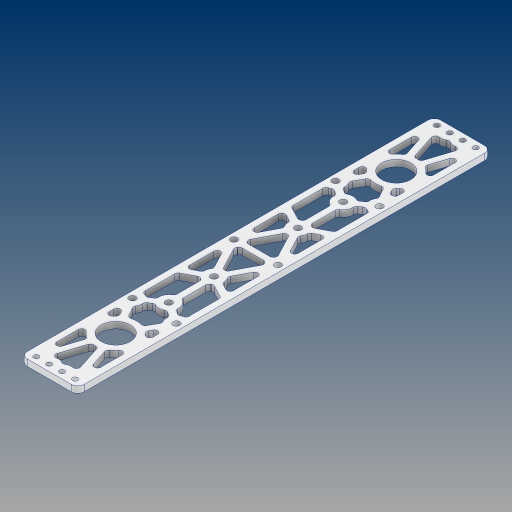
# Autodesk Inventor part: ELEV_019_SUPBAR3
Saved by Autodesk Inventor 2024.3 (Build 283343000, 343)
## iProperties
Created: 2024-11-28
Part Number: ELEV_019_SUPBAR3
Material: Aluminum 6061
Document SubType Name: Modeling
Designer: Kenji
Density: 2.7 g/cm^3
Appearance: Aluminum - Flat
Author: Kenji
Autodesk Inventor part; units mm, degrees
ref_plane "YZ Plane" through (0, 0, 0) normal (1, 0, 0) x (0, 1, 0)
ref_plane "XZ Plane" through (0, 0, 0) normal (0, 1, 0) x (-1, 0, 0)
ref_plane "XY Plane" through (0, 0, 0) normal (0, 0, 1) x (1, 0, 0)
sketch "Sketch1" plane through (0, 0, 0) normal (0, 1, 0) x (-1, 0, 0)
  line L0 (0, 0) -> (55.88, 0)
  line L1 (55.88, 0) -> (55.88, -406.4)
  line L2 (55.88, -406.4) -> (0, -406.4)
  line L3 (0, -406.4) -> (0, 0)
  circle A0 centre (27.94, -65.3034) radius 14.2875
  circle A1 centre (27.94, -341.0966) radius 14.2875
  line L4 (27.94, 0) -> (27.94, -406.4) construction
  circle A2 centre (27.94, -341.0966) radius 22.733 construction
  circle A3 centre (27.94, -65.3034) radius 22.733 construction
  circle A4 centre (27.94, -65.3034) radius 27.2288 construction
  circle A5 centre (27.94, -341.0966) radius 27.2288 construction
  circle A6 centre (27.94, -117.475) radius 3.2512
  circle A7 centre (27.94, -161.925) radius 3.2512
  circle A8 centre (27.94, -244.475) radius 3.2512
  circle A9 centre (27.94, -288.925) radius 3.2512
  line L5 (55.88, -203.2) -> (0, -203.2) construction
  line L6 (55.88, -368.3254) -> (0, -368.3254) construction
  line L7 (47.244, -254) -> (8.636, -254) construction
  line L8 (8.636, -254) -> (8.636, -279.4) construction
  line L9 (8.636, -279.4) -> (47.244, -279.4) construction
  line L10 (47.244, -279.4) -> (47.244, -254) construction
  line L11 (27.94, -254) -> (27.94, -279.4) construction
  circle A10 centre (8.89, -6.35) radius 2.54
  circle A11 centre (21.59, -6.35) radius 2.54
  circle A12 centre (34.29, -6.35) radius 2.54
  circle A13 centre (46.99, -6.35) radius 2.54
  circle A14 centre (8.89, -400.05) radius 2.54
  circle A15 centre (21.59, -400.05) radius 2.54
  circle A16 centre (34.29, -400.05) radius 2.54
  circle A17 centre (46.99, -400.05) radius 2.54
  circle A18 centre (49.53, -203.2) radius 3.2512
  circle A19 centre (49.53, -203.2) radius 6.35 construction
  circle A20 centre (6.35, -203.2) radius 3.2512
  circle A21 centre (6.35, -203.2) radius 6.35 construction
  line L12 (49.53, -203.2) -> (6.35, -203.2) construction
  circle A22 centre (49.53, -103.378) radius 3.2512
  circle A23 centre (6.35, -103.378) radius 3.2512
  circle A24 centre (49.53, -103.378) radius 6.35 construction
  circle A25 centre (6.35, -103.378) radius 6.35 construction
  line L13 (49.53, -103.378) -> (6.35, -103.378) construction
  line L14 (27.94, -103.378) -> (27.94, -92.5322) construction
  line L15 (27.94, -103.378) -> (27.94, -114.2238) construction
  circle A26 centre (49.53, -303.022) radius 3.2512
  circle A27 centre (6.35, -303.022) radius 3.2512
  point P0 (27.94, -266.7)
  dimension "d5" = 54.4576
  dimension "d0" = 55.88
  dimension "d1" = 406.4
  dimension "d2" = 28.575
  dimension "d4" = 45.466
  dimension "d6" = 6.5024
  dimension "d8" = 203.2
  dimension "d9" = 38.0746
  dimension "d10" = 44.45
  dimension "d15" = 25.4
  dimension "d16" = 38.608
  dimension "d17" = 19.304
  dimension "d18" = 9.525
  dimension "d19" = 12.7
  dimension "d20" = 139.7
  dimension "d31" = 5.08
  dimension "d34" = 12.7
  dimension "d39" = 8.89
  dimension "d40" = 6.35
  dimension "d47" = 6.5024
  dimension "d48" = 12.7
  constraints: 30 end point, 26 centre point, 10 equal radius, 8 coincident, 8 midpoint, 6 perpendicular, 6 symmetric about line, 5 tangent, 4 horizontal, 4 parallel, 2 collinear, 2 point on line, 2 vertical alignment, 1 vertical, 31 other
  measures "d0" distance between parallel lines of L3 L1
  measures "d1" distance between parallel lines of L2 L0
  measures "d2" diameter of A1
  measures "d4" diameter of A2
  measures "d6" diameter of A8
  measures "d8" distance between parallel lines of L0 L5
  measures "d9" distance between parallel lines of L2 L6
  measures "d10" distance of A9.centre A8.centre
  measures "d15" distance of L9.end L7.start
  measures "d16" distance of L7.start L7.end
  measures "d17" distance between parallel lines of L10 L11
  measures "d18" distance from line of A9.centre L9
  measures "d19" distance from line of L9 point (27.94, -266.7)
  measures "d20" distance from line of L2 point (27.94, -266.7)
  measures "d31" diameter of A10
  measures "d34" distance of A10.centre A11.centre
  measures "d39" distance from line of A13.centre L1
  measures "d40" distance from line of L0 A13.centre
  measures "d47" diameter of A18
  measures "d48" diameter of A19
extrude "Extrusion3" add sketch "Sketch1" along normal blind 6.35
fillet "Fillet6" radius 6.35 4 edges at (-55.88, 3.175, 0) (0, 3.175, 0) (-55.88, 3.175, -406.4) (0, 3.175, -406.4)
sketch "Sketch3" plane through (0, 6.35, 0) normal (0, 1, 0) x (1, 0, 0)
  arc A0 (0, 400.05) -> (-6.35, 406.4) centre (-6.35, 400.05) ccw construction
  line L0 (-6.35, 406.4) -> (-49.53, 406.4) construction
  arc A1 (-49.53, 406.4) -> (-55.88, 400.05) centre (-49.53, 400.05) ccw construction
  line L1 (-55.88, 400.05) -> (-55.88, 6.35) construction
  arc A2 (-55.88, 6.35) -> (-49.53, 0) centre (-49.53, 6.35) ccw construction
  line L2 (-49.53, 0) -> (-6.35, 0) construction
  arc A3 (-6.35, 0) -> (0, 6.35) centre (-6.35, 6.35) ccw construction
  line L3 (0, 6.35) -> (0, 400.05) construction
  circle A4 centre (-6.35, 303.022) radius 3.2512 construction
  circle A5 centre (-6.35, 103.378) radius 3.2512 construction
  circle A6 centre (-6.35, 203.2) radius 3.2512 construction
  circle A7 centre (-8.89, 400.05) radius 2.54 construction
  circle A8 centre (-34.29, 400.05) radius 2.54 construction
  circle A9 centre (-46.99, 6.35) radius 2.54 construction
  circle A10 centre (-21.59, 6.35) radius 2.54 construction
  circle A11 centre (-8.89, 6.35) radius 2.54 construction
  circle A12 centre (-27.94, 288.925) radius 3.2512 construction
  circle A13 centre (-27.94, 244.475) radius 3.2512 construction
  circle A14 centre (-27.94, 161.925) radius 3.2512 construction
  circle A15 centre (-27.94, 117.475) radius 3.2512 construction
  circle A16 centre (-27.94, 341.0966) radius 14.2875 construction
  circle A17 centre (-27.94, 65.3034) radius 14.2875 construction
  circle A18 centre (-34.29, 6.35) radius 2.54 construction
  circle A19 centre (-46.99, 400.05) radius 2.54 construction
  circle A20 centre (-21.59, 400.05) radius 2.54 construction
  circle A21 centre (-49.53, 203.2) radius 3.2512 construction
  circle A22 centre (-49.53, 103.378) radius 3.2512 construction
  circle A23 centre (-49.53, 303.022) radius 3.2512 construction
  line L4 (-49.53, 6.35) -> (-49.53, 400.05) construction
  line L5 (-49.53, 400.05) -> (-6.35, 400.05) construction
  line L6 (-6.35, 400.05) -> (-6.35, 6.35) construction
  line L7 (-6.35, 6.35) -> (-49.53, 6.35) construction
  circle A24 centre (-46.99, 6.35) radius 8.89 construction
  circle A25 centre (-34.29, 6.35) radius 8.89 construction
  circle A26 centre (-21.59, 6.35) radius 8.89 construction
  circle A27 centre (-8.89, 6.35) radius 8.89 construction
  circle A28 centre (-27.94, 65.3034) radius 20.6375 construction
  circle A29 centre (-49.53, 103.378) radius 9.6012 construction
  circle A30 centre (-27.94, 117.475) radius 9.6012 construction
  circle A31 centre (-6.35, 103.378) radius 9.6012 construction
  circle A32 centre (-27.94, 161.925) radius 9.6012 construction
  circle A33 centre (-49.53, 203.2) radius 9.6012 construction
  circle A34 centre (-6.35, 203.2) radius 9.6012 construction
  circle A35 centre (-27.94, 244.475) radius 9.6012 construction
  circle A36 centre (-49.53, 303.022) radius 9.6012 construction
  circle A37 centre (-27.94, 288.925) radius 9.6012 construction
  circle A38 centre (-6.35, 303.022) radius 9.6012 construction
  circle A39 centre (-46.99, 400.05) radius 8.89 construction
  circle A40 centre (-27.94, 341.0966) radius 20.6375 construction
  circle A41 centre (-34.29, 400.05) radius 8.89 construction
  circle A42 centre (-21.59, 400.05) radius 8.89 construction
  circle A43 centre (-8.89, 400.05) radius 8.89 construction
  line L8 (-41.4908, 108.6272) -> (-35.9792, 112.2258) construction
  line L9 (-19.9008, 112.2258) -> (-14.3892, 108.6272) construction
  line L10 (-17.7603, 83.2556) -> (-11.0859, 95.0261) construction
  line L11 (-49.53, 65.3034) -> (-48.5775, 65.3034) construction
  line L12 (-7.3025, 65.3034) -> (-6.35, 65.3034) construction
  line L13 (-34.2857, 45.6657) -> (-44.2565, 14.8093) construction
  line L14 (-11.6235, 14.8093) -> (-21.5943, 45.6657) construction
  line L15 (-44.7941, 95.0261) -> (-38.1197, 83.2556) construction
  line L16 (-41.2996, 95.3002) -> (-36.4986, 86.8335)
  line L17 (-38.5113, 106.7807) -> (-35.487, 108.7554)
  line L18 (-20.393, 108.7554) -> (-17.3687, 106.7807)
  line L19 (-19.3814, 86.8335) -> (-14.5804, 95.3002)
  arc A44 (-22.9162, 85.3201) -> (-32.9638, 85.3201) centre (-27.94, 65.3034) ccw
  arc A45 (-32.3071, 108.9245) -> (-23.5729, 108.9245) centre (-27.94, 117.475) ccw
  arc A46 (-36.4986, 86.8335) -> (-32.9638, 85.3201) centre (-33.7367, 88.3996) ccw
  arc A47 (-22.9162, 85.3201) -> (-19.3814, 86.8335) centre (-22.1433, 88.3996) ccw
  arc A48 (-20.393, 108.7554) -> (-23.5729, 108.9245) centre (-22.1288, 106.0969) ccw
  arc A49 (-32.3071, 108.9245) -> (-35.487, 108.7554) centre (-33.7512, 106.0969) ccw
  line L20 (-38.018, 44.4413) -> (-43.3338, 27.9905)
  line L21 (-49.53, 28.9667) -> (-49.53, 50.2063)
  arc A50 (-43.8997, 52.2192) -> (-39.2926, 48.069) centre (-27.94, 65.3034) ccw
  arc A51 (-38.018, 44.4413) -> (-39.2926, 48.069) centre (-41.0391, 45.4175) ccw
  arc A52 (-49.53, 28.9667) -> (-43.3338, 27.9905) centre (-46.355, 28.9667) ccw
  circle A53 centre (-46.355, 50.2063) radius 3.175 construction
  arc A54 (-43.8997, 52.2192) -> (-49.53, 50.2063) centre (-46.355, 50.2063) ccw
  line L22 (-12.5462, 27.9905) -> (-17.862, 44.4413)
  line L23 (-6.35, 50.2063) -> (-6.35, 28.9667)
  arc A55 (-16.5874, 48.069) -> (-11.9803, 52.2192) centre (-27.94, 65.3034) ccw
  arc A56 (-16.5874, 48.069) -> (-17.862, 44.4413) centre (-14.8409, 45.4175) ccw
  arc A57 (-12.5462, 27.9905) -> (-6.35, 28.9667) centre (-9.525, 28.9667) ccw
  circle A58 centre (-9.525, 50.2063) radius 3.175 construction
  arc A59 (-6.35, 50.2063) -> (-11.9803, 52.2192) centre (-9.525, 50.2063) ccw
  line L24 (-49.53, 80.4005) -> (-49.53, 84.9053)
  arc A60 (-42.5383, 79.8909) -> (-43.8997, 78.3876) centre (-27.94, 65.3034) ccw
  arc A61 (-41.2694, 98.4845) -> (-39.9451, 103.9373) centre (-49.53, 103.378) ccw
  arc A62 (-15.9349, 103.9373) -> (-14.6106, 98.4845) centre (-6.35, 103.378) ccw
  arc A63 (-14.5804, 95.3002) -> (-14.6106, 98.4845) centre (-17.3423, 96.8663) ccw
  arc A64 (-15.9349, 103.9373) -> (-17.3687, 106.7807) centre (-19.1045, 104.1222) ccw
  arc A65 (-38.5113, 106.7807) -> (-39.9451, 103.9373) centre (-36.7755, 104.1222) ccw
  arc A66 (-41.2694, 98.4845) -> (-41.2996, 95.3002) centre (-38.5377, 96.8663) ccw
  line L25 (-43.5931, 86.4714) -> (-42.0223, 83.7013)
  arc A67 (-43.5931, 86.4714) -> (-49.53, 84.9053) centre (-46.355, 84.9053) ccw
  arc A68 (-42.5383, 79.8909) -> (-42.0223, 83.7013) centre (-44.7842, 82.1352) ccw
  circle A69 centre (-46.355, 80.4005) radius 3.175 construction
  arc A70 (-49.53, 80.4005) -> (-43.8997, 78.3876) centre (-46.355, 80.4005) ccw
  line L26 (-31.9756, 42.4888) -> (-39.5042, 19.1903)
  line L27 (-16.3758, 19.1903) -> (-23.9044, 42.4888)
  arc A71 (-29.6111, 13.9091) -> (-35.9059, 15.0919) centre (-34.29, 6.35) ccw
  arc A72 (-19.9741, 15.0919) -> (-26.2689, 13.9091) centre (-21.59, 6.35) ccw
  arc A73 (-28.8192, 44.6846) -> (-27.0608, 44.6846) centre (-27.94, 65.3034) ccw
  arc A74 (-28.8192, 44.6846) -> (-31.9756, 42.4888) centre (-28.9544, 41.5125) ccw
  arc A75 (-23.9044, 42.4888) -> (-27.0608, 44.6846) centre (-26.9256, 41.5125) ccw
  arc A76 (-29.6111, 13.9091) -> (-26.2689, 13.9091) centre (-27.94, 16.6087) ccw
  circle A77 centre (-36.483, 18.214) radius 3.175 construction
  circle A78 centre (-19.397, 18.214) radius 3.175 construction
  arc A79 (-39.5042, 19.1903) -> (-35.9059, 15.0919) centre (-36.483, 18.214) ccw
  arc A80 (-19.9741, 15.0919) -> (-16.3758, 19.1903) centre (-19.397, 18.214) ccw
  line L28 (-13.8577, 83.7013) -> (-12.2869, 86.4714)
  line L29 (-6.35, 84.9053) -> (-6.35, 80.4005)
  arc A81 (-11.9803, 78.3876) -> (-13.3417, 79.8909) centre (-27.94, 65.3034) ccw
  arc A82 (-8.0576, 93.9299) -> (-6.35, 93.7768) centre (-6.35, 103.378) ccw
  arc A83 (-13.8577, 83.7013) -> (-13.3417, 79.8909) centre (-11.0958, 82.1352) ccw
  arc A84 (-6.35, 84.9053) -> (-12.2869, 86.4714) centre (-9.525, 84.9053) ccw
  circle A85 centre (-9.525, 80.4005) radius 3.175 construction
  arc A86 (-11.9803, 78.3876) -> (-6.35, 80.4005) centre (-9.525, 80.4005) ccw
  line L30 (-27.94, 127.0762) -> (-27.94, 152.3238) construction
  line L31 (-23.4899, 170.4326) -> (-10.8001, 194.6924) construction
  line L32 (-32.3901, 170.4326) -> (-45.0799, 194.6924) construction
  line L33 (-19.4324, 157.4749) -> (-6.35, 150.6318) construction
  line L34 (-36.4476, 157.4749) -> (-49.53, 150.6318) construction
  line L35 (-31.115, 128.5614) -> (-31.115, 150.8386)
  line L36 (-24.765, 128.5614) -> (-24.765, 150.8386)
  line L37 (-36.2921, 153.9731) -> (-47.8266, 147.9397)
  line L38 (-41.983, 112.0976) -> (-38.9587, 114.0723)
  line L39 (-49.53, 145.1263) -> (-49.53, 115.7534)
  arc A87 (-45.1629, 111.9285) -> (-47.144, 112.678) centre (-49.53, 103.378) ccw
  arc A88 (-32.712, 125.8063) -> (-37.5249, 116.9157) centre (-27.94, 117.475) ccw
  arc A89 (-33.1106, 153.835) -> (-32.712, 153.5937) centre (-27.94, 161.925) ccw
  arc A90 (-47.8266, 147.9397) -> (-49.53, 145.1263) centre (-46.355, 145.1263) ccw
  arc A91 (-33.1106, 153.835) -> (-36.2921, 153.9731) centre (-34.8205, 151.1597) ccw
  arc A92 (-31.115, 150.8386) -> (-32.712, 153.5937) centre (-34.29, 150.8386) ccw
  arc A93 (-32.712, 125.8063) -> (-31.115, 128.5614) centre (-34.29, 128.5614) ccw
  arc A94 (-38.9587, 114.0723) -> (-37.5249, 116.9157) centre (-40.6945, 116.7308) ccw
  arc A95 (-45.1629, 111.9285) -> (-41.983, 112.0976) centre (-43.7188, 114.7561) ccw
  arc A96 (-49.53, 115.7534) -> (-47.144, 112.678) centre (-46.355, 115.7534) ccw
  line L40 (-49.53, 203.2) -> (-6.35, 203.2) construction
  line L41 (-16.9213, 114.0723) -> (-13.897, 112.0976)
  line L42 (-19.5879, 153.9731) -> (-8.0534, 147.9397)
  line L43 (-6.35, 115.7534) -> (-6.35, 145.1263)
  arc A97 (-18.3551, 116.9157) -> (-23.168, 125.8063) centre (-27.94, 117.475) ccw
  arc A98 (-8.736, 112.678) -> (-10.7171, 111.9285) centre (-6.35, 103.378) ccw
  arc A99 (-23.168, 153.5937) -> (-22.7694, 153.835) centre (-27.94, 161.925) ccw
  arc A100 (-18.3551, 116.9157) -> (-16.9213, 114.0723) centre (-15.1855, 116.7308) ccw
  arc A101 (-8.736, 112.678) -> (-6.35, 115.7534) centre (-9.525, 115.7534) ccw
  arc A102 (-13.897, 112.0976) -> (-10.7171, 111.9285) centre (-12.1612, 114.7561) ccw
  arc A103 (-24.765, 128.5614) -> (-23.168, 125.8063) centre (-21.59, 128.5614) ccw
  arc A104 (-23.168, 153.5937) -> (-24.765, 150.8386) centre (-21.59, 150.8386) ccw
  arc A105 (-19.5879, 153.9731) -> (-22.7694, 153.835) centre (-21.0595, 151.1597) ccw
  arc A106 (-6.35, 145.1263) -> (-8.0534, 147.9397) centre (-9.525, 145.1263) ccw
  line L44 (-39.2353, 159.5998) -> (-44.8834, 156.6454)
  line L45 (-35.8919, 170.2771) -> (-43.5416, 184.9016)
  line L46 (-49.53, 159.4588) -> (-49.53, 183.43)
  arc A107 (-36.03, 167.0956) -> (-37.5342, 162.2919) centre (-27.94, 161.925) ccw
  arc A108 (-43.5416, 184.9016) -> (-49.53, 183.43) centre (-46.355, 183.43) ccw
  arc A109 (-49.53, 159.4588) -> (-44.8834, 156.6454) centre (-46.355, 159.4588) ccw
  arc A110 (-39.2353, 159.5998) -> (-37.5342, 162.2919) centre (-40.7069, 162.4132) ccw
  arc A111 (-36.03, 167.0956) -> (-35.8919, 170.2771) centre (-38.7053, 168.8055) ccw
  line L47 (-19.9881, 170.2771) -> (-12.3384, 184.9016)
  line L48 (-16.6447, 159.5998) -> (-10.9966, 156.6454)
  line L49 (-6.35, 159.4588) -> (-6.35, 183.43)
  arc A112 (-6.35, 183.43) -> (-12.3384, 184.9016) centre (-9.525, 183.43) ccw
  arc A113 (-10.9966, 156.6454) -> (-6.35, 159.4588) centre (-9.525, 159.4588) ccw
  arc A114 (-18.3458, 162.2919) -> (-19.85, 167.0956) centre (-27.94, 161.925) ccw
  arc A115 (-18.3458, 162.2919) -> (-16.6447, 159.5998) centre (-15.1731, 162.4132) ccw
  arc A116 (-19.9881, 170.2771) -> (-19.85, 167.0956) centre (-17.1747, 168.8055) ccw
  line L50 (-38.4436, 200.025) -> (-17.4364, 200.025)
  line L51 (-30.7534, 174.1536) -> (-41.5781, 194.8479)
  line L52 (-25.1266, 174.1536) -> (-14.3019, 194.8479)
  arc A117 (-30.7534, 174.1536) -> (-25.1266, 174.1536) centre (-27.94, 175.6252) ccw
  arc A118 (-41.44, 198.0294) -> (-41.1987, 198.428) centre (-49.53, 203.2) ccw
  arc A119 (-14.6813, 198.428) -> (-14.44, 198.0294) centre (-6.35, 203.2) ccw
  arc A120 (-41.44, 198.0294) -> (-41.5781, 194.8479) centre (-38.7647, 196.3195) ccw
  arc A121 (-38.4436, 200.025) -> (-41.1987, 198.428) centre (-38.4436, 196.85) ccw
  arc A122 (-14.6813, 198.428) -> (-17.4364, 200.025) centre (-17.4364, 196.85) ccw
  arc A123 (-14.3019, 194.8479) -> (-14.44, 198.0294) centre (-17.1153, 196.3195) ccw
  point P0 (0, 0)
  point P1 (-35.2366, 84.608)
  point P2 (-33.7911, 109.8627)
  point P3 (-22.0889, 109.8627)
  point P4 (-20.6434, 84.608)
  point P5 (-15.6728, 105.6734)
  point P6 (-13.5813, 97.0621)
  point P7 (-42.2987, 97.0621)
  point P8 (-40.2072, 105.6734)
  point P9 (-37.2313, 46.8758)
  point P10 (-49.53, 8.8154)
  point P11 (-6.35, 8.8154)
  point P12 (-18.6487, 46.8758)
  point P13 (-49.53, 93.7768)
  point P14 (-40.7604, 81.4757)
  point P15 (-47.8224, 93.9299)
  point P16 (-31.1889, 44.9232)
  point P17 (-24.6911, 44.9232)
  point P18 (-15.1196, 81.4757)
  point P19 (-31.115, 126.536)
  point P20 (-31.115, 152.864)
  point P21 (-24.765, 126.536)
  point P22 (-24.765, 152.864)
  point P23 (-34.4974, 154.9119)
  point P24 (-49.53, 147.0486)
  point P25 (-43.6789, 110.9903)
  point P26 (-37.2628, 115.1796)
  point P27 (-49.53, 112.9792)
  point P28 (-18.6172, 115.1796)
  point P29 (-12.2011, 110.9903)
  point P30 (-21.3826, 154.9119)
  point P31 (-6.35, 147.0486)
  point P32 (-6.35, 112.9792)
  point P33 (-37.4406, 160.5386)
  point P34 (-49.53, 154.2149)
  point P35 (-34.9531, 168.4824)
  point P36 (-48.1436, 193.6994)
  point P37 (-49.53, 193.5988)
  point P38 (-20.9269, 168.4824)
  point P39 (-7.7364, 193.6994)
  point P40 (-18.4394, 160.5386)
  point P41 (-6.35, 154.2149)
  point P42 (-6.35, 193.5988)
  point P43 (-40.469, 200.025)
  point P44 (-15.411, 200.025)
  point P45 (-29.3264, 171.4256)
  point P46 (-42.5169, 196.6426)
  point P47 (-26.5536, 171.4256)
  point P48 (-13.3631, 196.6426)
  dimension "d53" = 6.35
  dimension "d54" = 6.35
  dimension "d55" = 6.35
  dimension "d56" = 6.35
  dimension "d57" = 6.35
  dimension "d58" = 6.35
  dimension "d59" = 6.35
  dimension "d60" = 6.35
  dimension "d61" = 6.35
  dimension "d62" = 6.35
  dimension "d63" = 6.35
  dimension "d64" = 6.35
  dimension "d65" = 6.35
  dimension "d66" = 6.35
  dimension "d67" = 6.35
  dimension "d68" = 6.35
  dimension "d69" = 6.35
  dimension "d70" = 6.35
  dimension "d71" = 6.35
  dimension "d72" = 6.35
  dimension "d73" = 6.35
  dimension "d76" = 3.175
  dimension "d77" = 3.175
  dimension "d78" = 3.175
  dimension "d79" = 3.175
  dimension "d80" = 3.175
  dimension "d85" = 3.175
  dimension "d86" = 3.175
  dimension "d87" = 3.175
  dimension "d88" = 6.35
  dimension "d89" = 3.175
  dimension "d91" = 3.175
  dimension "d92" = 3.175
  dimension "d93" = 6.35
  dimension "d97" = 3.175
  dimension "d98" = 3.175
  dimension "d99" = 3.175
  dimension "d100" = 6.35
  dimension "d103" = 3.175
  dimension "d104" = 3.175
  dimension "d105" = 3.175
  dimension "d106" = 3.175
  dimension "d107" = 6.35
  dimension "d108" = 6.35
  dimension "d109" = 3.175
  dimension "d111" = 3.175
  dimension "d112" = 6.35
  dimension "d115" = 3.175
  dimension "d116" = 3.175
  dimension "d117" = 3.175
  dimension "d118" = 3.175
  dimension "d119" = 3.175
  dimension "d120" = 3.175
  dimension "d121" = 3.175
  dimension "d122" = 3.175
  dimension "d123" = 3.175
  dimension "d124" = 3.175
  dimension "d125" = 3.175
  dimension "d126" = 3.175
  dimension "d127" = 3.175
  dimension "d128" = 3.175
  dimension "d129" = 3.175
  dimension "d130" = 3.175
  dimension "d131" = 3.175
  constraints: 204 point on circle, 102 tangent, 94 end point, 91 centre point, 77 point on line, 26 equal radius, 23 parallel, 6 vertical, 4 concentric, 3 horizontal, 2 perpendicular, 141 other
  measures "d63" radial gap between concentric circles of A21 A33
  measures "d64" radial gap between concentric circles of A6 A34
  measures "d65" radial gap between concentric circles of A13 A35
  measures "d66" radial gap between concentric circles of A23 A36
  measures "d67" radial gap between concentric circles of A12 A37
  measures "d68" radial gap between concentric circles of A4 A38
  measures "d69" radial gap between concentric circles of A19 A39
  measures "d70" radial gap between concentric circles of A16 A40
  measures "d71" radial gap between concentric circles of A8 A41
  measures "d72" radial gap between concentric circles of A20 A42
  measures "d73" radial gap between concentric circles of A7 A43
  measures "d76" distance between parallel lines of L15 L16
  measures "d77" distance between parallel lines of L8 L17
  measures "d78" distance between parallel lines of L9 L18
  measures "d79" distance between parallel lines of L10 L19
  measures "d80" radius of A46
  measures "d85" distance between parallel lines of L13 L20
  measures "d86" radius of A51
  measures "d87" radius of A52
  measures "d88" diameter of A53
  measures "d89" distance between parallel lines of L14 L22
  measures "d91" radius of A56
  measures "d92" radius of A57
  measures "d93" diameter of A58
  measures "d97" radius of A63
  measures "d98" distance between parallel lines of L15 L25
  measures "d99" radius of A67
  measures "d100" diameter of A69
  measures "d103" distance between parallel lines of L13 L26
  measures "d104" distance between parallel lines of L14 L27
  measures "d105" radius of A74
  measures "d106" radius of A76
  measures "d107" diameter of A77
  measures "d108" diameter of A78
  measures "d109" distance between parallel lines of L10 L28
  measures "d111" radius of A83
  measures "d112" diameter of A85
  measures "d115" distance between parallel lines of L30 L35
  measures "d116" distance between parallel lines of L30 L36
  measures "d117" distance between parallel lines of L34 L37
  measures "d118" distance between parallel lines of L8 L38
  measures "d119" radius of A90
  measures "d120" distance between parallel lines of L9 L41
  measures "d121" distance between parallel lines of L33 L42
  measures "d122" radius of A100
  measures "d123" radius of A101
  measures "d124" distance between parallel lines of L34 L44
  measures "d125" distance between parallel lines of L32 L45
  measures "d126" radius of A108
  measures "d127" radius of A109
  measures "d128" radius of A110
  measures "d129" distance between parallel lines of L31 L47
  measures "d130" distance between parallel lines of L33 L48
  measures "d131" radius of A112
extrude "Extrusion4" cut sketch "Sketch3" against normal blind 6.35
sketch "Sketch4" plane through (0, 6.35, 0) normal (0, 1, 0) x (1, 0, 0)
  arc A0 (-10.9966, 156.6454) -> (-6.35, 159.4588) centre (-9.525, 159.4588) ccw projected
  line L0 (-10.9966, 156.6454) -> (-16.6447, 159.5998) projected
  arc A1 (-18.3458, 162.2919) -> (-16.6447, 159.5998) centre (-15.1731, 162.4132) ccw projected
  arc A2 (-18.3458, 162.2919) -> (-19.85, 167.0956) centre (-27.94, 161.925) ccw projected
  arc A3 (-19.9881, 170.2771) -> (-19.85, 167.0956) centre (-17.1747, 168.8055) ccw projected
  line L1 (-19.9881, 170.2771) -> (-12.3384, 184.9016) projected
  arc A4 (-6.35, 183.43) -> (-12.3384, 184.9016) centre (-9.525, 183.43) ccw projected
  line L2 (-6.35, 183.43) -> (-6.35, 159.4588) projected
  arc A5 (-6.35, 84.9053) -> (-12.2869, 86.4714) centre (-9.525, 84.9053) ccw projected
  line L3 (-6.35, 84.9053) -> (-6.35, 80.4005) projected
  arc A6 (-11.9803, 78.3876) -> (-6.35, 80.4005) centre (-9.525, 80.4005) ccw projected
  arc A7 (-11.9803, 78.3876) -> (-13.3417, 79.8909) centre (-27.94, 65.3034) ccw projected
  arc A8 (-13.8577, 83.7013) -> (-13.3417, 79.8909) centre (-11.0958, 82.1352) ccw projected
  line L4 (-13.8577, 83.7013) -> (-12.2869, 86.4714) projected
  arc A9 (-16.5874, 48.069) -> (-17.862, 44.4413) centre (-14.8409, 45.4175) ccw projected
  arc A10 (-16.5874, 48.069) -> (-11.9803, 52.2192) centre (-27.94, 65.3034) ccw projected
  arc A11 (-6.35, 50.2063) -> (-11.9803, 52.2192) centre (-9.525, 50.2063) ccw projected
  line L5 (-6.35, 50.2063) -> (-6.35, 28.9667) projected
  arc A12 (-12.5462, 27.9905) -> (-6.35, 28.9667) centre (-9.525, 28.9667) ccw projected
  line L6 (-12.5462, 27.9905) -> (-17.862, 44.4413) projected
  arc A13 (-43.5931, 86.4714) -> (-49.53, 84.9053) centre (-46.355, 84.9053) ccw projected
  line L7 (-43.5931, 86.4714) -> (-42.0223, 83.7013) projected
  arc A14 (-42.5383, 79.8909) -> (-42.0223, 83.7013) centre (-44.7842, 82.1352) ccw projected
  arc A15 (-42.5383, 79.8909) -> (-43.8997, 78.3876) centre (-27.94, 65.3034) ccw projected
  arc A16 (-49.53, 80.4005) -> (-43.8997, 78.3876) centre (-46.355, 80.4005) ccw projected
  line L8 (-49.53, 80.4005) -> (-49.53, 84.9053) projected
  arc A17 (-31.115, 150.8386) -> (-32.712, 153.5937) centre (-34.29, 150.8386) ccw projected
  line L9 (-31.115, 150.8386) -> (-31.115, 128.5614) projected
  arc A18 (-32.712, 125.8063) -> (-31.115, 128.5614) centre (-34.29, 128.5614) ccw projected
  arc A19 (-32.712, 125.8063) -> (-37.5249, 116.9157) centre (-27.94, 117.475) ccw projected
  arc A20 (-38.9587, 114.0723) -> (-37.5249, 116.9157) centre (-40.6945, 116.7308) ccw projected
  line L10 (-38.9587, 114.0723) -> (-41.983, 112.0976) projected
  arc A21 (-45.1629, 111.9285) -> (-41.983, 112.0976) centre (-43.7188, 114.7561) ccw projected
  arc A22 (-45.1629, 111.9285) -> (-47.144, 112.678) centre (-49.53, 103.378) ccw projected
  arc A23 (-49.53, 115.7534) -> (-47.144, 112.678) centre (-46.355, 115.7534) ccw projected
  line L11 (-49.53, 115.7534) -> (-49.53, 145.1263) projected
  arc A24 (-47.8266, 147.9397) -> (-49.53, 145.1263) centre (-46.355, 145.1263) ccw projected
  line L12 (-47.8266, 147.9397) -> (-36.2921, 153.9731) projected
  arc A25 (-33.1106, 153.835) -> (-36.2921, 153.9731) centre (-34.8205, 151.1597) ccw projected
  arc A26 (-33.1106, 153.835) -> (-32.712, 153.5937) centre (-27.94, 161.925) ccw projected
  arc A27 (-30.7534, 174.1536) -> (-25.1266, 174.1536) centre (-27.94, 175.6252) ccw projected
  line L13 (-30.7534, 174.1536) -> (-41.5781, 194.8479) projected
  arc A28 (-41.44, 198.0294) -> (-41.5781, 194.8479) centre (-38.7647, 196.3195) ccw projected
  arc A29 (-41.44, 198.0294) -> (-41.1987, 198.428) centre (-49.53, 203.2) ccw projected
  arc A30 (-38.4436, 200.025) -> (-41.1987, 198.428) centre (-38.4436, 196.85) ccw projected
  line L14 (-38.4436, 200.025) -> (-17.4364, 200.025) projected
  arc A31 (-14.6813, 198.428) -> (-17.4364, 200.025) centre (-17.4364, 196.85) ccw projected
  arc A32 (-14.6813, 198.428) -> (-14.44, 198.0294) centre (-6.35, 203.2) ccw projected
  arc A33 (-14.3019, 194.8479) -> (-14.44, 198.0294) centre (-17.1153, 196.3195) ccw projected
  line L15 (-14.3019, 194.8479) -> (-25.1266, 174.1536) projected
  arc A34 (-36.4986, 86.8335) -> (-32.9638, 85.3201) centre (-33.7367, 88.3996) ccw projected
  line L16 (-36.4986, 86.8335) -> (-41.2996, 95.3002) projected
  arc A35 (-41.2694, 98.4845) -> (-41.2996, 95.3002) centre (-38.5377, 96.8663) ccw projected
  arc A36 (-41.2694, 98.4845) -> (-39.9451, 103.9373) centre (-49.53, 103.378) ccw projected
  arc A37 (-38.5113, 106.7807) -> (-39.9451, 103.9373) centre (-36.7755, 104.1222) ccw projected
  line L17 (-38.5113, 106.7807) -> (-35.487, 108.7554) projected
  arc A38 (-32.3071, 108.9245) -> (-35.487, 108.7554) centre (-33.7512, 106.0969) ccw projected
  arc A39 (-32.3071, 108.9245) -> (-23.5729, 108.9245) centre (-27.94, 117.475) ccw projected
  arc A40 (-20.393, 108.7554) -> (-23.5729, 108.9245) centre (-22.1288, 106.0969) ccw projected
  line L18 (-20.393, 108.7554) -> (-17.3687, 106.7807) projected
  arc A41 (-15.9349, 103.9373) -> (-17.3687, 106.7807) centre (-19.1045, 104.1222) ccw projected
  arc A42 (-15.9349, 103.9373) -> (-14.6106, 98.4845) centre (-6.35, 103.378) ccw projected
  arc A43 (-14.5804, 95.3002) -> (-14.6106, 98.4845) centre (-17.3423, 96.8663) ccw projected
  line L19 (-14.5804, 95.3002) -> (-19.3814, 86.8335) projected
  arc A44 (-22.9162, 85.3201) -> (-19.3814, 86.8335) centre (-22.1433, 88.3996) ccw projected
  arc A45 (-22.9162, 85.3201) -> (-32.9638, 85.3201) centre (-27.94, 65.3034) ccw projected
  arc A46 (-39.5042, 19.1903) -> (-35.9059, 15.0919) centre (-36.483, 18.214) ccw projected
  line L20 (-39.5042, 19.1903) -> (-31.9756, 42.4888) projected
  arc A47 (-28.8192, 44.6846) -> (-31.9756, 42.4888) centre (-28.9544, 41.5125) ccw projected
  arc A48 (-28.8192, 44.6846) -> (-27.0608, 44.6846) centre (-27.94, 65.3034) ccw projected
  arc A49 (-23.9044, 42.4888) -> (-27.0608, 44.6846) centre (-26.9256, 41.5125) ccw projected
  line L21 (-23.9044, 42.4888) -> (-16.3758, 19.1903) projected
  arc A50 (-19.9741, 15.0919) -> (-16.3758, 19.1903) centre (-19.397, 18.214) ccw projected
  arc A51 (-19.9741, 15.0919) -> (-26.2689, 13.9091) centre (-21.59, 6.35) ccw projected
  arc A52 (-29.6111, 13.9091) -> (-26.2689, 13.9091) centre (-27.94, 16.6087) ccw projected
  arc A53 (-29.6111, 13.9091) -> (-35.9059, 15.0919) centre (-34.29, 6.35) ccw projected
  arc A54 (-49.53, 28.9667) -> (-43.3338, 27.9905) centre (-46.355, 28.9667) ccw projected
  line L22 (-49.53, 28.9667) -> (-49.53, 50.2063) projected
  arc A55 (-43.8997, 52.2192) -> (-49.53, 50.2063) centre (-46.355, 50.2063) ccw projected
  arc A56 (-43.8997, 52.2192) -> (-39.2926, 48.069) centre (-27.94, 65.3034) ccw projected
  arc A57 (-38.018, 44.4413) -> (-39.2926, 48.069) centre (-41.0391, 45.4175) ccw projected
  line L23 (-38.018, 44.4413) -> (-43.3338, 27.9905) projected
  arc A58 (-13.897, 112.0976) -> (-10.7171, 111.9285) centre (-12.1612, 114.7561) ccw projected
  line L24 (-13.897, 112.0976) -> (-16.9213, 114.0723) projected
  arc A59 (-18.3551, 116.9157) -> (-16.9213, 114.0723) centre (-15.1855, 116.7308) ccw projected
  arc A60 (-18.3551, 116.9157) -> (-23.168, 125.8063) centre (-27.94, 117.475) ccw projected
  arc A61 (-24.765, 128.5614) -> (-23.168, 125.8063) centre (-21.59, 128.5614) ccw projected
  line L25 (-24.765, 128.5614) -> (-24.765, 150.8386) projected
  arc A62 (-23.168, 153.5937) -> (-24.765, 150.8386) centre (-21.59, 150.8386) ccw projected
  arc A63 (-23.168, 153.5937) -> (-22.7694, 153.835) centre (-27.94, 161.925) ccw projected
  arc A64 (-19.5879, 153.9731) -> (-22.7694, 153.835) centre (-21.0595, 151.1597) ccw projected
  line L26 (-19.5879, 153.9731) -> (-8.0534, 147.9397) projected
  arc A65 (-6.35, 145.1263) -> (-8.0534, 147.9397) centre (-9.525, 145.1263) ccw projected
  line L27 (-6.35, 145.1263) -> (-6.35, 115.7534) projected
  arc A66 (-8.736, 112.678) -> (-6.35, 115.7534) centre (-9.525, 115.7534) ccw projected
  arc A67 (-8.736, 112.678) -> (-10.7171, 111.9285) centre (-6.35, 103.378) ccw projected
  arc A68 (-43.5416, 184.9016) -> (-49.53, 183.43) centre (-46.355, 183.43) ccw projected
  line L28 (-43.5416, 184.9016) -> (-35.8919, 170.2771) projected
  arc A69 (-36.03, 167.0956) -> (-35.8919, 170.2771) centre (-38.7053, 168.8055) ccw projected
  arc A70 (-36.03, 167.0956) -> (-37.5342, 162.2919) centre (-27.94, 161.925) ccw projected
  arc A71 (-39.2353, 159.5998) -> (-37.5342, 162.2919) centre (-40.7069, 162.4132) ccw projected
  line L29 (-39.2353, 159.5998) -> (-44.8834, 156.6454) projected
  arc A72 (-49.53, 159.4588) -> (-44.8834, 156.6454) centre (-46.355, 159.4588) ccw projected
  line L30 (-49.53, 159.4588) -> (-49.53, 183.43) projected
  arc A73 (0, 400.05) -> (-6.35, 406.4) centre (-6.35, 400.05) ccw projected
  line L31 (-6.35, 406.4) -> (-49.53, 406.4) projected
  arc A74 (-49.53, 406.4) -> (-55.88, 400.05) centre (-49.53, 400.05) ccw projected
  line L32 (-55.88, 400.05) -> (-55.88, 6.35) projected
  arc A75 (-55.88, 6.35) -> (-49.53, 0) centre (-49.53, 6.35) ccw projected
  line L33 (-49.53, 0) -> (-6.35, 0) projected
  arc A76 (-6.35, 0) -> (0, 6.35) centre (-6.35, 6.35) ccw projected
  line L34 (0, 6.35) -> (0, 400.05) projected
  circle A77 centre (-6.35, 303.022) radius 3.2512 projected
  circle A78 centre (-6.35, 103.378) radius 3.2512 projected
  circle A79 centre (-6.35, 203.2) radius 3.2512 projected
  circle A80 centre (-8.89, 400.05) radius 2.54 projected
  circle A81 centre (-34.29, 400.05) radius 2.54 projected
  circle A82 centre (-46.99, 6.35) radius 2.54 projected
  circle A83 centre (-21.59, 6.35) radius 2.54 projected
  circle A84 centre (-8.89, 6.35) radius 2.54 projected
  circle A85 centre (-27.94, 288.925) radius 3.2512 projected
  circle A86 centre (-27.94, 244.475) radius 3.2512 projected
  circle A87 centre (-27.94, 161.925) radius 3.2512 projected
  circle A88 centre (-27.94, 117.475) radius 3.2512 projected
  circle A89 centre (-27.94, 341.0966) radius 14.2875 projected
  circle A90 centre (-27.94, 65.3034) radius 14.2875 projected
  circle A91 centre (-34.29, 6.35) radius 2.54 projected
  circle A92 centre (-46.99, 400.05) radius 2.54 projected
  circle A93 centre (-21.59, 400.05) radius 2.54 projected
  circle A94 centre (-49.53, 203.2) radius 3.2512 projected
  circle A95 centre (-49.53, 103.378) radius 3.2512 projected
  circle A96 centre (-49.53, 303.022) radius 3.2512 projected
  line L35 (-49.53, 203.2) -> (-6.35, 203.2) construction
  arc A97 (-6.35, 246.9412) -> (-10.9966, 249.7546) centre (-9.525, 246.9412) ccw
  line L36 (-10.9966, 249.7546) -> (-16.6447, 246.8002)
  arc A98 (-16.6447, 246.8002) -> (-18.3458, 244.1081) centre (-15.1731, 243.9868) ccw
  arc A99 (-19.85, 239.3044) -> (-18.3458, 244.1081) centre (-27.94, 244.475) ccw
  arc A100 (-19.85, 239.3044) -> (-19.9881, 236.1229) centre (-17.1747, 237.5945) ccw
  line L37 (-19.9881, 236.1229) -> (-12.3384, 221.4984)
  arc A101 (-12.3384, 221.4984) -> (-6.35, 222.97) centre (-9.525, 222.97) ccw
  line L38 (-6.35, 222.97) -> (-6.35, 246.9412)
  arc A102 (-12.2869, 319.9286) -> (-6.35, 321.4947) centre (-9.525, 321.4947) ccw
  line L39 (-6.35, 321.4947) -> (-6.35, 325.9995)
  arc A103 (-6.35, 325.9995) -> (-11.9803, 328.0124) centre (-9.525, 325.9995) ccw
  arc A104 (-13.3417, 326.5091) -> (-11.9803, 328.0124) centre (-27.94, 341.0966) ccw
  arc A105 (-13.3417, 326.5091) -> (-13.8577, 322.6987) centre (-11.0958, 324.2648) ccw
  line L40 (-13.8577, 322.6987) -> (-12.2869, 319.9286)
  arc A106 (-17.862, 361.9587) -> (-16.5874, 358.331) centre (-14.8409, 360.9825) ccw
  arc A107 (-11.9803, 354.1808) -> (-16.5874, 358.331) centre (-27.94, 341.0966) ccw
  arc A108 (-11.9803, 354.1808) -> (-6.35, 356.1937) centre (-9.525, 356.1937) ccw
  line L41 (-6.35, 356.1937) -> (-6.35, 377.4333)
  arc A109 (-6.35, 377.4333) -> (-12.5462, 378.4095) centre (-9.525, 377.4333) ccw
  line L42 (-12.5462, 378.4095) -> (-17.862, 361.9587)
  arc A110 (-49.53, 321.4947) -> (-43.5931, 319.9286) centre (-46.355, 321.4947) ccw
  line L43 (-43.5931, 319.9286) -> (-42.0223, 322.6987)
  arc A111 (-42.0223, 322.6987) -> (-42.5383, 326.5091) centre (-44.7842, 324.2648) ccw
  arc A112 (-43.8997, 328.0124) -> (-42.5383, 326.5091) centre (-27.94, 341.0966) ccw
  arc A113 (-43.8997, 328.0124) -> (-49.53, 325.9995) centre (-46.355, 325.9995) ccw
  line L44 (-49.53, 325.9995) -> (-49.53, 321.4947)
  arc A114 (-32.712, 252.8063) -> (-31.115, 255.5614) centre (-34.29, 255.5614) ccw
  line L45 (-31.115, 255.5614) -> (-31.115, 277.8386)
  arc A115 (-31.115, 277.8386) -> (-32.712, 280.5937) centre (-34.29, 277.8386) ccw
  arc A116 (-37.5249, 289.4843) -> (-32.712, 280.5937) centre (-27.94, 288.925) ccw
  arc A117 (-37.5249, 289.4843) -> (-38.9587, 292.3277) centre (-40.6945, 289.6692) ccw
  line L46 (-38.9587, 292.3277) -> (-41.983, 294.3024)
  arc A118 (-41.983, 294.3024) -> (-45.1629, 294.4715) centre (-43.7188, 291.6439) ccw
  arc A119 (-47.144, 293.722) -> (-45.1629, 294.4715) centre (-49.53, 303.022) ccw
  arc A120 (-47.144, 293.722) -> (-49.53, 290.6466) centre (-46.355, 290.6466) ccw
  line L47 (-49.53, 290.6466) -> (-49.53, 261.2737)
  arc A121 (-49.53, 261.2737) -> (-47.8266, 258.4603) centre (-46.355, 261.2737) ccw
  line L48 (-47.8266, 258.4603) -> (-36.2921, 252.4269)
  arc A122 (-36.2921, 252.4269) -> (-33.1106, 252.565) centre (-34.8205, 255.2403) ccw
  arc A123 (-32.712, 252.8063) -> (-33.1106, 252.565) centre (-27.94, 244.475) ccw
  arc A124 (-25.1266, 232.2464) -> (-30.7534, 232.2464) centre (-27.94, 230.7748) ccw
  line L49 (-30.7534, 232.2464) -> (-41.5781, 211.5521)
  arc A125 (-41.5781, 211.5521) -> (-41.44, 208.3706) centre (-38.7647, 210.0805) ccw
  arc A126 (-41.1987, 207.972) -> (-41.44, 208.3706) centre (-49.53, 203.2) ccw
  arc A127 (-41.1987, 207.972) -> (-38.4436, 206.375) centre (-38.4436, 209.55) ccw
  line L50 (-38.4436, 206.375) -> (-17.4364, 206.375)
  arc A128 (-17.4364, 206.375) -> (-14.6813, 207.972) centre (-17.4364, 209.55) ccw
  arc A129 (-14.44, 208.3706) -> (-14.6813, 207.972) centre (-6.35, 203.2) ccw
  arc A130 (-14.44, 208.3706) -> (-14.3019, 211.5521) centre (-17.1153, 210.0805) ccw
  line L51 (-14.3019, 211.5521) -> (-25.1266, 232.2464)
  arc A131 (-32.9638, 321.0799) -> (-36.4986, 319.5665) centre (-33.7367, 318.0004) ccw
  line L52 (-36.4986, 319.5665) -> (-41.2996, 311.0998)
  arc A132 (-41.2996, 311.0998) -> (-41.2694, 307.9155) centre (-38.5377, 309.5337) ccw
  arc A133 (-39.9451, 302.4627) -> (-41.2694, 307.9155) centre (-49.53, 303.022) ccw
  arc A134 (-39.9451, 302.4627) -> (-38.5113, 299.6193) centre (-36.7755, 302.2778) ccw
  line L53 (-38.5113, 299.6193) -> (-35.487, 297.6446)
  arc A135 (-35.487, 297.6446) -> (-32.3071, 297.4755) centre (-33.7512, 300.3031) ccw
  arc A136 (-23.5729, 297.4755) -> (-32.3071, 297.4755) centre (-27.94, 288.925) ccw
  arc A137 (-23.5729, 297.4755) -> (-20.393, 297.6446) centre (-22.1288, 300.3031) ccw
  line L54 (-20.393, 297.6446) -> (-17.3687, 299.6193)
  arc A138 (-17.3687, 299.6193) -> (-15.9349, 302.4627) centre (-19.1045, 302.2778) ccw
  arc A139 (-14.6106, 307.9155) -> (-15.9349, 302.4627) centre (-6.35, 303.022) ccw
  arc A140 (-14.6106, 307.9155) -> (-14.5804, 311.0998) centre (-17.3423, 309.5337) ccw
  line L55 (-14.5804, 311.0998) -> (-19.3814, 319.5665)
  arc A141 (-19.3814, 319.5665) -> (-22.9162, 321.0799) centre (-22.1433, 318.0004) ccw
  arc A142 (-32.9638, 321.0799) -> (-22.9162, 321.0799) centre (-27.94, 341.0966) ccw
  arc A143 (-35.9059, 391.3081) -> (-39.5042, 387.2097) centre (-36.483, 388.186) ccw
  line L56 (-39.5042, 387.2097) -> (-31.9756, 363.9112)
  arc A144 (-31.9756, 363.9112) -> (-28.8192, 361.7154) centre (-28.9544, 364.8875) ccw
  arc A145 (-27.0608, 361.7154) -> (-28.8192, 361.7154) centre (-27.94, 341.0966) ccw
  arc A146 (-27.0608, 361.7154) -> (-23.9044, 363.9112) centre (-26.9256, 364.8875) ccw
  line L57 (-23.9044, 363.9112) -> (-16.3758, 387.2097)
  arc A147 (-16.3758, 387.2097) -> (-19.9741, 391.3081) centre (-19.397, 388.186) ccw
  arc A148 (-26.2689, 392.4909) -> (-19.9741, 391.3081) centre (-21.59, 400.05) ccw
  arc A149 (-26.2689, 392.4909) -> (-29.6111, 392.4909) centre (-27.94, 389.7913) ccw
  arc A150 (-35.9059, 391.3081) -> (-29.6111, 392.4909) centre (-34.29, 400.05) ccw
  arc A151 (-43.3338, 378.4095) -> (-49.53, 377.4333) centre (-46.355, 377.4333) ccw
  line L58 (-49.53, 377.4333) -> (-49.53, 356.1937)
  arc A152 (-49.53, 356.1937) -> (-43.8997, 354.1808) centre (-46.355, 356.1937) ccw
  arc A153 (-39.2926, 358.331) -> (-43.8997, 354.1808) centre (-27.94, 341.0966) ccw
  arc A154 (-39.2926, 358.331) -> (-38.018, 361.9587) centre (-41.0391, 360.9825) ccw
  line L59 (-38.018, 361.9587) -> (-43.3338, 378.4095)
  arc A155 (-10.7171, 294.4715) -> (-13.897, 294.3024) centre (-12.1612, 291.6439) ccw
  line L60 (-13.897, 294.3024) -> (-16.9213, 292.3277)
  arc A156 (-16.9213, 292.3277) -> (-18.3551, 289.4843) centre (-15.1855, 289.6692) ccw
  arc A157 (-23.168, 280.5937) -> (-18.3551, 289.4843) centre (-27.94, 288.925) ccw
  arc A158 (-23.168, 280.5937) -> (-24.765, 277.8386) centre (-21.59, 277.8386) ccw
  line L61 (-24.765, 277.8386) -> (-24.765, 255.5614)
  arc A159 (-24.765, 255.5614) -> (-23.168, 252.8063) centre (-21.59, 255.5614) ccw
  arc A160 (-22.7694, 252.565) -> (-23.168, 252.8063) centre (-27.94, 244.475) ccw
  arc A161 (-22.7694, 252.565) -> (-19.5879, 252.4269) centre (-21.0595, 255.2403) ccw
  line L62 (-19.5879, 252.4269) -> (-8.0534, 258.4603)
  arc A162 (-8.0534, 258.4603) -> (-6.35, 261.2737) centre (-9.525, 261.2737) ccw
  line L63 (-6.35, 261.2737) -> (-6.35, 290.6466)
  arc A163 (-6.35, 290.6466) -> (-8.736, 293.722) centre (-9.525, 290.6466) ccw
  arc A164 (-10.7171, 294.4715) -> (-8.736, 293.722) centre (-6.35, 303.022) ccw
  arc A165 (-49.53, 222.97) -> (-43.5416, 221.4984) centre (-46.355, 222.97) ccw
  line L64 (-43.5416, 221.4984) -> (-35.8919, 236.1229)
  arc A166 (-35.8919, 236.1229) -> (-36.03, 239.3044) centre (-38.7053, 237.5945) ccw
  arc A167 (-37.5342, 244.1081) -> (-36.03, 239.3044) centre (-27.94, 244.475) ccw
  arc A168 (-37.5342, 244.1081) -> (-39.2353, 246.8002) centre (-40.7069, 243.9868) ccw
  line L65 (-39.2353, 246.8002) -> (-44.8834, 249.7546)
  arc A169 (-44.8834, 249.7546) -> (-49.53, 246.9412) centre (-46.355, 246.9412) ccw
  line L66 (-49.53, 246.9412) -> (-49.53, 222.97)
  arc A170 (-49.53, 406.4) -> (-55.88, 400.05) centre (-49.53, 400.05) ccw
  line L67 (-49.53, 406.4) -> (-6.35, 406.4)
  arc A171 (0, 400.05) -> (-6.35, 406.4) centre (-6.35, 400.05) ccw
  circle A172 centre (-6.35, 303.022) radius 3.2512
  circle A173 centre (-46.99, 400.05) radius 2.54
  circle A174 centre (-21.59, 400.05) radius 2.54
  circle A175 centre (-8.89, 400.05) radius 2.54
  circle A176 centre (-27.94, 244.475) radius 3.2512
  circle A177 centre (-27.94, 288.925) radius 3.2512
  circle A178 centre (-27.94, 341.0966) radius 14.2875
  circle A179 centre (-34.29, 400.05) radius 2.54
  circle A180 centre (-49.53, 303.022) radius 3.2512
  point P0 (0, 0)
  point P1 (0, 406.4)
  constraints: 187 symmetric about line, 150 point on circle, 84 centre point, 66 end point, 1 horizontal, 84 other
extrude "Extrusion5" cut sketch "Sketch4" against normal blind 6.35 contours L38 A101 L37 A100 A99 A98 L36 A97 | L40 A105 A104 A103 L39 A102 | L42 A109 L41 A108 A107 A106 | L44 A113 A112 A111 L43 A110 | A123 A122 L48 A121 L47 A120 A119 A118 L46 A117 A116 A115 L45 A114 | L51 A130 A129 A128 L50 A127 A126 A125 L49 A124 | A142 A141 L55 A140 A139 A138 L54 A137 A136 A135 L53 A134 A133 A132 L52 A131 | A150 A149 A148 A147 L57 A146 A145 A144 L56 A143 | L59 A154 A153 A152 L58 A151 | A164 A163 L63 A162 L62 A161 A160 A159 L61 A158 A157 A156 L60 A155 | L66 A169 L65 A168 A167 A166 L64 A165
equation "\"d17\" = 0.5 * d16"
body "Solid3"
